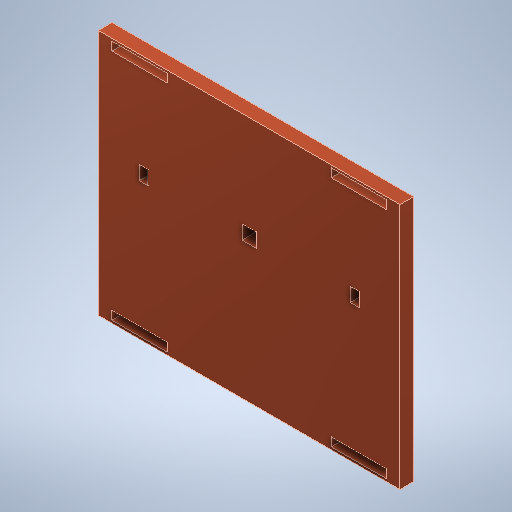
# Autodesk Inventor part: chassis arriere
Saved by Autodesk Inventor 2026.2 (Build 302298010, 298A)
## iProperties
Created: 2026-03-16
Part Number: chassis arriere
Material: Générique
Document SubType Name: Modeling
Designer: genon
Density: 1 g/cm^3
Appearance: Cuivre - Satiné
Author: genon
Autodesk Inventor part; units mm, degrees
ref_plane "YZ Plane" through (0, 0, 0) normal (1, 0, 0) x (0, 1, 0)
ref_plane "XZ Plane" through (0, 0, 0) normal (0, 1, 0) x (-1, 0, 0)
ref_plane "XY Plane" through (0, 0, 0) normal (0, 0, 1) x (1, 0, 0)
sketch "Esquisse1" plane through (0, 0, 0) normal (0, 0, 1) x (1, 0, 0)
  line L0 (0, 0) -> (100, 0)
  line L1 (100, 0) -> (100, 80)
  line L2 (100, 80) -> (0, 80)
  line L3 (0, 80) -> (0, 0)
  dimension "d0" = 100
  dimension "d1" = 80
  constraints: 8 end point, 2 parallel, 1 horizontal, 1 perpendicular
  measures "d0" distance of L2.end L1.end
  measures "d1" distance of L1.end L0.end
extrude "Extrusion1" add sketch "Esquisse1" against normal blind 5
sketch "Esquisse7" plane through (0, 0, 0) normal (0, 0, 1) x (1, 0, 0)
  line L0 (0, 0) -> (0, 45)
  line L1 (0, 0) -> (0, 80) projected
  line L2 (0, 45) -> (100, 45)
  line L3 (50, 45) -> (10, 45)
  line L4 (50, 45) -> (90, 45)
  line L5 (10, 45) -> (13, 45)
  line L6 (13, 45) -> (13, 50)
  line L7 (13, 50) -> (10, 50)
  line L8 (10, 50) -> (10, 45)
  line L9 (90, 45) -> (87, 45)
  line L10 (87, 45) -> (87, 50)
  line L11 (87, 50) -> (90, 50)
  line L12 (90, 50) -> (90, 45)
  line L13 (50, 45) -> (52.5, 45)
  line L14 (52.5, 45) -> (52.5, 50)
  line L15 (52.5, 50) -> (47.5, 50)
  line L16 (47.5, 50) -> (47.5, 45)
  line L17 (50, 45) -> (47.5, 45)
  line L18 (86.9, 44.9) -> (90.1, 44.9)
  line L19 (90.1, 44.9) -> (90.1, 50.1)
  line L20 (90.1, 50.1) -> (86.9, 50.1)
  line L21 (86.9, 50.1) -> (86.9, 44.9)
  line L22 (86.9, 44.9) -> (90.1, 50.1) construction
  line L23 (90.1, 44.9) -> (86.9, 50.1) construction
  line L24 (47.4, 44.9) -> (52.6, 44.9)
  line L25 (52.6, 44.9) -> (52.6, 50.1)
  line L26 (52.6, 50.1) -> (47.4, 50.1)
  line L27 (47.4, 50.1) -> (47.4, 44.9)
  line L28 (47.4, 44.9) -> (52.6, 50.1) construction
  line L29 (52.6, 44.9) -> (47.4, 50.1) construction
  line L30 (9.9, 44.9) -> (13.1, 44.9)
  line L31 (13.1, 44.9) -> (13.1, 50.1)
  line L32 (13.1, 50.1) -> (9.9, 50.1)
  line L33 (9.9, 50.1) -> (9.9, 44.9)
  line L34 (9.9, 44.9) -> (13.1, 50.1) construction
  line L35 (13.1, 44.9) -> (9.9, 50.1) construction
  point P0 (87, 45)
  point P1 (13, 45)
  point P2 (52.5, 45)
  point P3 (88.5, 47.5)
  point P4 (50, 47.5)
  point P5 (11.5, 47.5)
  point P6 (90.1, 45)
  point P7 (86.9, 45)
  point P8 (52.6, 45)
  point P9 (47.4, 45)
  point P10 (13.1, 45)
  point P11 (9.9, 45)
  dimension "d42" = 45
  dimension "d43" = 100
  dimension "d44" = 40
  dimension "d45" = 40
  dimension "d46" = 3
  dimension "d47" = 5
  dimension "d48" = 3
  dimension "d49" = 5
  dimension "d53" = 2.5
  dimension "d54" = 5
  dimension "d55" = 5
  dimension "d56" = 3.2
  dimension "d57" = 5.2
  dimension "d58" = 5.2
  dimension "d59" = 3.2
  dimension "d60" = 5.2
  dimension "d61" = 5.2
  constraints: 70 end point, 10 parallel, 9 perpendicular, 7 midpoint, 6 point on line, 5 horizontal, 1 collinear
  measures "d42" distance of L0.start L0.end
  measures "d43" distance of L0.end L2.end
  measures "d44" distance of L3.start L3.end
  measures "d45" distance of L3.start L4.end
  measures "d46" distance of L7.end L6.end
  measures "d47" distance of L6.end L5.end
  measures "d48" distance of L10.end L11.end
  measures "d49" distance of L9.end L10.end
  measures "d53" distance of L3.start L13.end
  measures "d54" distance of L13.end L14.end
  measures "d55" distance of L14.end L15.end
  measures "d56" distance of L20.end L19.end
  measures "d57" distance of L19.end L18.end
  measures "d58" distance of L26.end L25.end
  measures "d59" distance of L32.end L31.end
  measures "d60" distance of L31.end L30.end
  measures "d61" distance between parallel lines of L24 L26
extrude "Extrusion2" cut sketch "Esquisse7" against normal through all contours L8 L7 L6 L2 | L2 L33 L32 L31 L6 L7 L8 | L16 L15 L14 L2 | L2 L27 L26 L25 L14 L15 L16 | L10 L11 L12 L2 | L2 L21 L20 L19 L12 L11 L10
sketch "Esquisse8" plane through (0, 0, 0) normal (0, 0, 1) x (1, 0, 0)
  line L0 (0, 0) -> (0, 40)
  line L1 (0, 0) -> (0, 80) projected
  line L2 (0, 40) -> (50, 40)
  line L3 (100, 80) -> (100, 0) projected
  line L4 (-5, -5) -> (105, -5)
  line L5 (105, -5) -> (105, 85)
  line L6 (105, 85) -> (-5, 85)
  line L7 (-5, 85) -> (-5, -5)
  line L8 (-5, -5) -> (105, 85) construction
  line L9 (105, -5) -> (-5, 85) construction
  line L10 (100, 80) -> (0, 80) projected
  line L11 (0, 80) -> (0, 0) projected
  line L12 (0, 0) -> (100, 0) projected
  line L13 (100, 0) -> (100, 80) projected
  dimension "d62" = 40
  dimension "d63" = 50
  dimension "d64" = 110
  dimension "d65" = 90
  constraints: 16 end point, 3 midpoint, 2 parallel, 2 perpendicular, 1 horizontal
  measures "d62" distance of L0.start L0.end
  measures "d63" distance of L0.end L2.end
  measures "d64" distance of L6.end L5.end
  measures "d65" distance of L5.end L4.end
extrude "Extrusion3" add sketch "Esquisse8" against normal blind 5
sketch "Esquisse9" plane through (0, 0, 0) normal (0, 0, 1) x (1, 0, 0)
  line L0 (0, 0) -> (-0.05, 0)
  line L1 (-0.05, 0) -> (-0.05, -0.95)
  line L2 (-0.05, -0.95) -> (20.05, -0.95)
  line L3 (20.05, -0.95) -> (20.05, -4.05)
  line L4 (20.05, -4.05) -> (-0.05, -4.05)
  line L5 (-0.05, -4.05) -> (-0.05, -0.95)
  line L6 (-5, -5) -> (105, -5) projected
  line L7 (105, -5) -> (50, -5)
  line L8 (50, -5) -> (50, 40.0521)
  line L9 (-5, -5) -> (-5, 85) projected
  line L10 (-5, 85) -> (-5, 40)
  line L11 (-5, 40) -> (20.05, 40)
  line L12 (100.05, -0.95) -> (79.95, -0.95)
  line L13 (79.95, -0.95) -> (79.95, -4.05)
  line L14 (79.95, -4.05) -> (100.05, -4.05)
  line L15 (100.05, -4.05) -> (100.05, -0.95)
  line L16 (-0.05, 80.95) -> (20.05, 80.95)
  line L17 (20.05, 80.95) -> (20.05, 84.05)
  line L18 (20.05, 84.05) -> (-0.05, 84.05)
  line L19 (-0.05, 84.05) -> (-0.05, 80.95)
  line L20 (100.05, 80.95) -> (79.95, 80.95)
  line L21 (79.95, 84.05) -> (100.05, 84.05)
  line L22 (79.95, 80.95) -> (79.95, 84.05)
  line L23 (100.05, 84.05) -> (100.05, 80.95)
  dimension "d68" = 0.05
  dimension "d69" = 0.95
  dimension "d70" = 20.1
  dimension "d71" = 3.1
  dimension "d72" = 55
  dimension "d73" = 45
  constraints: 44 end point, 12 symmetric about line, 4 perpendicular, 2 horizontal, 2 midpoint, 2 parallel
  measures "d68" distance of L0.start L0.end
  measures "d69" distance of L0.end L1.end
  measures "d70" distance of L3.end L4.end
  measures "d71" distance of L2.end L3.end
  measures "d72" distance of L6.end L7.end
  measures "d73" distance of L9.end L10.end
extrude "Extrusion4" cut sketch "Esquisse9" against normal blind 5
